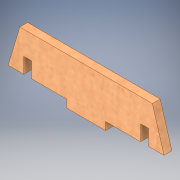
# Autodesk Inventor part: Limiter2
Saved by Autodesk Inventor 2019 (Build 230136000, 136)
## iProperties
Created: 2021-01-03
Part Number: Limiter2
Material: Дерево (вишня)
Document SubType Name: Modeling
Designer: Professional
Density: 0.63 g/cm^3
Appearance: Вишневое дерево — натуральный — со слабым глянцем
Author: Professional
Autodesk Inventor part; units mm, degrees
ref_plane "YZ Plane" through (0, 0, 0) normal (1, 0, 0) x (0, 1, 0)
ref_plane "XZ Plane" through (0, 0, 0) normal (0, 1, 0) x (-1, 0, 0)
ref_plane "XY Plane" through (0, 0, 0) normal (0, 0, 1) x (1, 0, 0)
sketch "Эскиз1" plane through (0, 0, 0) normal (0, 0, 1) x (1, 0, 0)
  line L0 (0, 0) -> (-10, 0)
  line L1 (-10, 0) -> (-10, 4)
  line L2 (-10, 4) -> (-28, 4)
  line L3 (-28, 4) -> (-28, 12)
  line L4 (-28, 12) -> (-32, 12)
  line L5 (-32, 12) -> (-32, 24) construction
  line L6 (-32, 24) -> (0, 24)
  line L7 (0, 24) -> (0, 0)
  line L8 (-32, 12) -> (-32, 4)
  line L9 (-32, 4) -> (-40, 4)
  line L10 (-40, 4) -> (-34, 24)
  line L11 (-34, 24) -> (-32, 24)
  line L12 (0, 0) -> (10, 0)
  line L13 (10, 0) -> (10, 4)
  line L14 (10, 4) -> (28, 4)
  line L15 (28, 4) -> (28, 12)
  line L16 (28, 12) -> (32, 12)
  line L17 (32, 12) -> (32, 24) construction
  line L18 (32, 24) -> (0, 24)
  line L19 (32, 12) -> (32, 4)
  line L20 (32, 4) -> (40, 4)
  line L21 (40, 4) -> (34, 24)
  line L22 (34, 24) -> (32, 24)
  dimension "d0" = 4
  dimension "d1" = 20
  dimension "d2" = 56
  dimension "d3" = 8
  dimension "d4" = 20
  dimension "d5" = 2
  dimension "d6" = 8
  constraints: 46 end point, 9 perpendicular, 9 symmetric about line, 2 point on line, 1 horizontal, 1 horizontal alignment, 1 parallel, 1 vertical
  measures "d0" distance of L0.end L1.end
  measures "d1" diameter of L1 L7
  measures "d2" diameter of L3 L7
  measures "d3" distance between parallel lines of L4 L2
  measures "d4" distance between parallel lines of L2 L6
  measures "d5" distance of L5.end L10.end
  measures "d6" distance of L8.end L9.end
extrude "Выдавливание1" add sketch "Эскиз1" along normal blind 4
